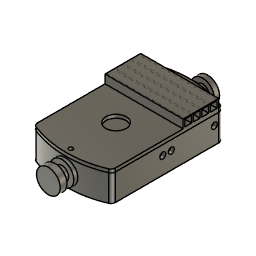
Case (Autodesk Fusion 360 design; units mm, degrees)
Autodesk Fusion 360 part; units mm, degrees
note: some values were not read from the file. Set by a fixed rule: which sketch regions a step uses.
sketch "Boceto1" plane through (0, 0, 0) normal (0, 0, 1) x (1, 0, 0)
  circle A0 centre (-5.9, 16.8256) radius 0.6
  line L0 (10.4, -15.2481) -> (-10.4, -15.2481)
  line L1 (-10.4, 15.5519) -> (-4.2071, 15.5519)
  circle A1 centre (5.9, 16.8256) radius 0.6
  spline S0 degree 3 poles (10.7171, -16.1976) (9.0911, -16.9299) (7.3492, -17.4466) (3.7858, -18.1418) (1.8989, -18.3158) (-4.1389, -18.2732) (-7.7725, -17.3263) (-10.6417, -16.2266) knots -1.732785 -1.732785 -1.732785 -1.732785 -1.337909 -1.337909 -0.921833 -0.921833 0 0 0 0
  line L2 (4.1929, 15.5519) -> (10.4, 15.5519)
  circle A2 centre (0, -16.6178) radius 0.6
  arc A3 (10.7171, -16.1976) -> (11.5, -15.0181) centre (10.22, -15.0181) ccw
  arc A4 (-11.5, -15.0181) -> (-10.6417, -16.2266) centre (-10.22, -15.0181) ccw
  line L3 (10.4, 15.5519) -> (10.4, -15.2481)
  line L4 (11.5, -15.0181) -> (11.4989, 15.4432)
  line L5 (-11.5011, 15.4432) -> (-11.5, -15.0181)
  line L6 (-10.4, -15.2481) -> (-10.4, 15.5519)
  line L7 (4.1929, 15.5519) -> (-4.2071, 15.5519)
  spline S1 degree 3 poles (-10.7181, 16.6227) (-9.0922, 17.355) (-7.3503, 17.8717) (-3.7869, 18.5669) (-1.9, 18.7409) (4.1378, 18.6983) (7.7714, 17.7514) (10.6407, 16.6517) knots -1.732785 -1.732785 -1.732785 -1.732785 -1.337909 -1.337909 -0.921833 -0.921833 0 0 0 0
  arc A5 (11.4989, 15.4432) -> (10.6407, 16.6517) centre (10.2189, 15.4432) ccw
  arc A6 (-10.7181, 16.6227) -> (-11.5011, 15.4432) centre (-10.2211, 15.4432) ccw
  point P0 (10.3989, 15.6732)
  point P1 (-10.4011, 15.6732)
  constraint coincident L5.start A6.end
  constraint coincident L4.end A5.start
extrude "Extruir1" add sketch "Boceto1" along normal blind 5.6 makes body 1
sketch "Boceto3" plane through (0, 0, 0) normal (0, 0, 1) x (1, 0, 0)
  spline S0 degree 3 poles (-10.7181, 16.6227) (-9.0922, 17.355) (-7.3503, 17.8717) (-3.7869, 18.5669) (-1.9, 18.7409) (4.1378, 18.6983) (7.7714, 17.7514) (10.6407, 16.6517) knots -1.732785 -1.732785 -1.732785 -1.732785 -1.337909 -1.337909 -0.921833 -0.921833 0 0 0 0
  line L0 (-11.5011, 15.4432) -> (-11.5, -15.0181)
  line L1 (11.5, -15.0181) -> (11.4989, 15.4432)
  spline S1 degree 3 poles (10.7171, -16.1976) (9.0911, -16.9299) (7.3492, -17.4466) (3.7858, -18.1418) (1.8989, -18.3158) (-4.1389, -18.2732) (-7.7725, -17.3263) (-10.6417, -16.2266) knots -1.732785 -1.732785 -1.732785 -1.732785 -1.337909 -1.337909 -0.921833 -0.921833 0 0 0 0
  arc A0 (-11.5, -15.0181) -> (-10.6417, -16.2266) centre (-10.22, -15.0181) ccw
  arc A1 (10.7171, -16.1976) -> (11.5, -15.0181) centre (10.22, -15.0181) ccw
  arc A2 (11.4989, 15.4432) -> (10.6407, 16.6517) centre (10.2189, 15.4432) ccw
  arc A3 (-10.7181, 16.6227) -> (-11.5011, 15.4432) centre (-10.2211, 15.4432) ccw
  point P0 (10.3989, 15.6732)
  point P1 (-10.4011, 15.6732)
  constraint coincident L0.start A3.end
  constraint coincident L1.end A2.start
extrude "Extruir2" add sketch "Boceto3" against normal blind 2.2 bodies 1
sketch "Boceto4" plane through (0, 0, 5.6) normal (0, 0, 1) x (-1, 0, 0)
  circle A0 centre (0, 16.6178) radius 0.6
  circle A1 centre (-5.9, -16.8256) radius 0.6
  circle A2 centre (5.9, -16.8256) radius 0.6
  line L0 (10.4, -15.5519) -> (-10.4, -15.5519)
  line L1 (-10.4, -15.5519) -> (-10.4, 15.2481)
  line L2 (-10.4, 15.2481) -> (10.4, 15.2481)
  line L3 (10.4, 15.2481) -> (10.4, -15.5519)
  arc A3 (-10.7171, 16.1976) -> (-11.5, 15.0181) centre (-10.22, 15.0181) ccw
  line L4 (-11.5, 15.0181) -> (-11.4989, -15.4432)
  line L5 (11.5011, -15.4432) -> (11.5, 15.0181)
  arc A4 (11.5, 15.0181) -> (10.6417, 16.2266) centre (10.22, 15.0181) ccw
  spline S0 degree 3 poles (10.6417, 16.2266) (7.7725, 17.3263) (4.1389, 18.2732) (-1.8989, 18.3158) (-3.7858, 18.1418) (-7.3492, 17.4466) (-9.0911, 16.9299) (-10.7171, 16.1976) knots 0 0 0 0 0.921833 0.921833 1.337909 1.337909 1.732785 1.732785 1.732785 1.732785
  line L6 (0, 16.6178) -> (0, 18.3024) construction
  line L7 (0, 18.3024) -> (0, 23.3024) construction
  line L8 (0, 23.3024) -> (5.4941, 23.3024) construction
  line L9 (0, -15.5519) -> (0, -18.7081) construction
  line L10 (0, -18.7081) -> (0, -23.7081) construction
  line L11 (0, -23.7081) -> (4.3514, -23.7081) construction
  arc A5 (-11.4989, -15.4432) -> (-10.6407, -16.6517) centre (-10.2189, -15.4432) ccw
  spline S1 degree 3 poles (-10.6407, -16.6517) (-7.7714, -17.7514) (-4.1378, -18.6983) (1.9, -18.7409) (3.7869, -18.5669) (7.3503, -17.8717) (9.0922, -17.355) (10.7181, -16.6227) knots 0 0 0 0 0.921833 0.921833 1.337909 1.337909 1.732785 1.732785 1.732785 1.732785
  arc A6 (10.7181, -16.6227) -> (11.5011, -15.4432) centre (10.2211, -15.4432) ccw
  dimension "d6" = 5
  dimension "d7" = 5
  constraint coincident A0.centre L6.start
  constraint coincident S0 L6.end
  constraint vertical L6
  constraint parallel L6 L7
  constraint perpendicular L7 L8
  constraint midpoint L0 L9.start
  constraint perpendicular L0 L9
  constraint perpendicular L0 L10
  constraint perpendicular L10 L11
  measures "d6" distance of L6.end L7.end
  measures "d7" distance of L9.end L10.end
ref_plane "PlanoDeObra1" through (-2.747, -23.3024, 5.6) normal (0, 1, 0) x (-1, 0, 0)
ref_plane "PlanoDeObra2" through (-2.1757, 23.7081, 5.6) normal (0, 1, 0) x (-1, 0, 0)
sketch "Boceto5" plane through (0, -23.3024, 0) normal (0, 1, 0) x (1, 0, 0)
  line L0 (10.7171, 2.2) -> (10.7171, -5.6)
  line L1 (-10.6417, -5.6) -> (10.7171, -5.6)
  line L2 (-10.6417, -5.6) -> (-10.6417, 2.2)
  line L3 (10.7171, 2.2) -> (-10.6417, 2.2)
  line L4 (-10.6417, -5.6) -> (10.7171, 2.2) construction
  line L5 (-10.6417, 2.2) -> (10.7171, -5.6) construction
  circle A0 centre (0.0377, -1.7) radius 3.5
  dimension "d10" = 7
  constraint coincident L1.start L2.start
  constraint coincident L0.start L3.start
  constraint coincident L2.end L3.end
  constraint coincident L0.end L1.end
  constraint midpoint L4 A0.centre
  measures "d10" diameter of A0
extrude "Extruir3" add sketch "Boceto5" along normal up to surface contours A0 end surface at (-2.3988, -18.1819, 2.4889) on bodies 1 bodies 1
sketch "Boceto6" plane through (0, 23.7081, 0) normal (0, 1, 0) x (1, 0, 0)
  line L0 (4.1929, 0) -> (-4.2071, 2.2) construction
  line L1 (4.1929, 2.2) -> (-4.2071, 0) construction
  line L2 (-10.7181, 2.2) -> (-10.7181, -5.6)
  line L3 (10.6407, -5.6) -> (-10.7181, -5.6)
  line L4 (10.6407, -5.6) -> (10.6407, 2.2)
  line L5 (-10.7181, 2.2) -> (10.6407, 2.2)
  line L6 (10.6407, -5.6) -> (-10.7181, 2.2) construction
  line L7 (10.6407, 2.2) -> (-10.7181, -5.6) construction
  circle A0 centre (-0.0387, -1.7) radius 3.5
  dimension "d42" = 7
  constraint coincident L3.start L4.start
  constraint coincident L2.start L5.start
  constraint coincident L4.end L5.end
  constraint coincident L2.end L3.end
  constraint midpoint L6 A0.centre
  measures "d42" diameter of A0
extrude "Extruir4" add sketch "Boceto6" against normal up to surface (8.1561 mm away) contours A0 bodies 1
sketch "Boceto7" plane through (0, 0, -2.2) normal (0, 0, -1) x (1, 0, 0)
  line L0 (11.4989, -15.4432) -> (11.5, 15.0181)
  arc A0 (11.5, 15.0181) -> (10.7171, 16.1976) centre (10.22, 15.0181) ccw
  spline S0 degree 3 poles (10.7171, 16.1976) (9.0911, 16.9299) (7.3492, 17.4466) (3.7858, 18.1418) (1.8989, 18.3158) (-4.1389, 18.2732) (-7.7725, 17.3263) (-10.6417, 16.2266) knots -1.732785 -1.732785 -1.732785 -1.732785 -1.337909 -1.337909 -0.921833 -0.921833 0 0 0 0
  arc A1 (-10.6417, 16.2266) -> (-11.5, 15.0181) centre (-10.22, 15.0181) ccw
  line L1 (-11.5, 15.0181) -> (-11.5011, -15.4432)
  arc A2 (-5.775, -6.6) -> (-5.775, -15) centre (-5.775, -10.8) ccw
  line L2 (5.775, 4.2) -> (-5.775, 4.2)
  arc A3 (5.775, -4.2) -> (5.775, 4.2) centre (5.775, 0) ccw
  arc A4 (5.775, -15) -> (5.775, -6.6) centre (5.775, -10.8) ccw
  line L3 (5.775, 15) -> (-5.775, 15)
  arc A5 (5.775, 6.6) -> (5.775, 15) centre (5.775, 10.8) ccw
  line L4 (-5.775, -15) -> (5.775, -15)
  arc A6 (-5.775, 4.2) -> (-5.775, -4.2) centre (-5.775, 0) ccw
  line L5 (-5.775, 6.6) -> (5.775, 6.6)
  arc A7 (-5.775, 15) -> (-5.775, 6.6) centre (-5.775, 10.8) ccw
  line L6 (-5.775, -4.2) -> (5.775, -4.2)
  line L7 (5.775, -6.6) -> (-5.775, -6.6)
  arc A8 (-11.5011, -15.4432) -> (-10.7181, -16.6227) centre (-10.2211, -15.4432) ccw
  spline S1 degree 3 poles (-10.7181, -16.6227) (-9.0922, -17.355) (-7.3503, -17.8717) (-3.7869, -18.5669) (-1.9, -18.7409) (4.1378, -18.6983) (7.7714, -17.7514) (10.6407, -16.6517) knots -1.732785 -1.732785 -1.732785 -1.732785 -1.337909 -1.337909 -0.921833 -0.921833 0 0 0 0
  arc A9 (10.6407, -16.6517) -> (11.4989, -15.4432) centre (10.2189, -15.4432) ccw
sketch "Boceto8" plane through (0, 0, 0) normal (0, 0, 1) x (-1, 0, 0)
  line L0 (10.4, -15.5519) -> (10.4, 15.2481)
  line L1 (10.4, 15.2481) -> (-10.4, 15.2481)
  line L2 (-10.4, 15.2481) -> (-10.4, -15.5519)
  line L3 (-10.4, -15.5519) -> (10.4, -15.5519)
  arc A0 (-1, 1.0002) -> (-1, -0.9998) centre (-1, 0.0002) ccw
  line L4 (3, 1.0002) -> (3, 1.0002)
  arc A1 (-1, 1.0002) -> (-1, -0.9998) centre (-1, 0.0002) ccw
  line L5 (-1, 11.7998) -> (3, 11.7998)
  line L6 (3, -11.7997) -> (-1, -11.7997)
  arc A2 (-1, -9.7997) -> (-1, -11.7997) centre (-1, -10.7997) ccw
  arc A3 (3, 9.7998) -> (3, 11.7998) centre (3, 10.7998) ccw
  arc A4 (3, -0.9998) -> (3, 1.0002) centre (3, 0.0002) ccw
  line L7 (-1, -11.7997) -> (3, -11.7997)
  line L8 (3, 9.7998) -> (-1, 9.7998)
  line L9 (-1, -0.9998) -> (3, -0.9998)
  arc A5 (3, -11.7997) -> (3, -9.7997) centre (3, -10.7997) ccw
  line L10 (3, -0.9998) -> (-1, -0.9998)
  line L11 (3, -9.7997) -> (-1, -9.7997)
  arc A6 (-1, 11.7998) -> (-1, 9.7998) centre (-1, 10.7998) ccw
  arc A7 (3, -0.9998) -> (3, 1.0002) centre (3, 0.0002) ccw
  arc A8 (3, -11.7997) -> (3, -9.7997) centre (3, -10.7997) ccw
  line L12 (-1, 1.0002) -> (3, 1.0002)
  arc A9 (-1, -9.7997) -> (-1, -11.7997) centre (-1, -10.7997) ccw
  line L13 (-1, 0.8945) -> (-1, 0.8945)
  line L14 (-1, 1.8945) -> (-1, 1.8945)
  line L15 (3, 1.8945) -> (3, 1.8945)
  line L16 (-1, -9.7997) -> (3, -9.7997)
  line L17 (3, 0.8945) -> (3, 0.8945)
extrude "Extruir5" cut sketch "Boceto8" against normal blind 1 contours A0 A1 A4 L9 L10 A7 L12 | L5 A3 L8 A6 | L6 A2 L7 A5 L11 A8 A9 L16 bodies 1
extrude "Extruir6" cut sketch "Boceto7" against normal blind 1.2 contours A2 A4 L4 L7 | L2 A3 A6 L6 | L3 A5 L5 A7 bodies 1
ref_plane "PlanoDeObra3" through (-0.0005, 0.2126, 5.6) normal (0, 0, 1) x (1, 0, 0)
sketch "Boceto9" plane through (0, 0, 5.6) normal (0, 0, 1) x (1, 0, 0)
  arc A0 (-10.7181, 16.6227) -> (-11.5011, 15.4432) centre (-10.2211, 15.4432) ccw
  arc A1 (11.4989, 15.4432) -> (10.6407, 16.6517) centre (10.2189, 15.4432) ccw
  line L0 (-10.4, 15.5519) -> (-4.2071, 15.5519)
  line L1 (-11.5011, 15.4432) -> (-11.5, -15.0181)
  circle A2 centre (-5.9, 16.8256) radius 0.6
  arc A3 (10.7171, -16.1976) -> (11.5, -15.0181) centre (10.22, -15.0181) ccw
  line L2 (11.5, -15.0181) -> (11.4989, 15.4432)
  spline S0 degree 3 poles (-10.7181, 16.6227) (-9.0922, 17.355) (-7.3503, 17.8717) (-3.7869, 18.5669) (-1.9, 18.7409) (4.1378, 18.6983) (7.7714, 17.7514) (10.6407, 16.6517) knots -1.732785 -1.732785 -1.732785 -1.732785 -1.337909 -1.337909 -0.921833 -0.921833 0 0 0 0
  line L3 (10.4, 15.5519) -> (10.4, -15.2481)
  circle A4 centre (0, -16.6178) radius 0.6
  line L4 (4.1929, 15.5519) -> (10.4, 15.5519)
  line L5 (-10.4, -15.2481) -> (-10.4, 15.5519)
  line L6 (4.1929, 15.5519) -> (-4.2071, 15.5519)
  spline S1 degree 3 poles (10.7171, -16.1976) (9.0911, -16.9299) (7.3492, -17.4466) (3.7858, -18.1418) (1.8989, -18.3158) (-4.1389, -18.2732) (-7.7725, -17.3263) (-10.6417, -16.2266) knots -1.732785 -1.732785 -1.732785 -1.732785 -1.337909 -1.337909 -0.921833 -0.921833 0 0 0 0
  arc A5 (-11.5, -15.0181) -> (-10.6417, -16.2266) centre (-10.22, -15.0181) ccw
  line L7 (10.4, -15.2481) -> (-10.4, -15.2481)
  circle A6 centre (5.9, 16.8256) radius 0.6
  point P0 (10.3989, 15.6732)
  point P1 (-10.4011, 15.6732)
  constraint coincident A0.end L1.start
  constraint coincident A1.start L2.end
extrude "Extruir7" add sketch "Boceto9" along normal blind 1 separate body contours A0 A1 L1 A3 L2 S0 S1 A5 | L0 L3 L4 L5 L6 L7 makes body 2
sketch "Boceto10" plane through (0, 0, 6.6) normal (0, 0, 1) x (-1, 0, 0)
  circle A0 centre (-5.9, -16.8256) radius 0.6
  circle A1 centre (0, 16.6178) radius 0.6
  circle A2 centre (5.9, -16.8256) radius 0.6
  arc A3 (10.7181, -16.6227) -> (11.5011, -15.4432) centre (10.2211, -15.4432) ccw
  line L0 (11.5011, -15.4432) -> (11.5, 15.0181)
  arc A4 (11.5, 15.0181) -> (10.6417, 16.2266) centre (10.22, 15.0181) ccw
  spline S0 degree 3 poles (10.6417, 16.2266) (7.7725, 17.3263) (4.1389, 18.2732) (-1.8989, 18.3158) (-3.7858, 18.1418) (-7.3492, 17.4466) (-9.0911, 16.9299) (-10.7171, 16.1976) knots 0 0 0 0 0.921833 0.921833 1.337909 1.337909 1.732785 1.732785 1.732785 1.732785
  arc A5 (-10.7171, 16.1976) -> (-11.5, 15.0181) centre (-10.22, 15.0181) ccw
  line L1 (-11.5, 15.0181) -> (-11.4989, -15.4432)
  arc A6 (-11.4989, -15.4432) -> (-10.6407, -16.6517) centre (-10.2189, -15.4432) ccw
  spline S1 degree 3 poles (-10.6407, -16.6517) (-7.7714, -17.7514) (-4.1378, -18.6983) (1.9, -18.7409) (3.7869, -18.5669) (7.3503, -17.8717) (9.0922, -17.355) (10.7181, -16.6227) knots 0 0 0 0 0.921833 0.921833 1.337909 1.337909 1.732785 1.732785 1.732785 1.732785
  line L2 (0, 16.6178) -> (0, 3.3178) construction
  circle A7 centre (0, 3.3178) radius 3
  dimension "d43" = 13.3
  dimension "d44" = 6
  constraint coincident A1.centre L2.start
  constraint vertical L2
  constraint coincident L2.end A7.centre
  measures "d43" distance of A1.centre L2.end
  measures "d44" diameter of A7
extrude "Extruir8" cut sketch "Boceto10" against normal through all contours A7 bodies 2
sketch "Boceto11" plane through (11.4995, 0.0004, 0) normal (1, 0.000035, 0) x (-0.000035, 1, 0)
  line L0 (-15.0185, 5.6) -> (-15.0185, -2.2)
  line L1 (-15.0185, -2.2) -> (15.4428, -2.2)
  line L2 (15.4428, -2.2) -> (15.4428, 0) construction
  line L3 (15.4428, 0) -> (-15.0185, 0) construction
  line L4 (-15.0185, 5.6) -> (15.4428, 0) construction
  line L5 (-15.0185, 0) -> (15.4219, 5.6) construction
  line L6 (0.2122, 2.8) -> (0.2122, 0) construction
  line L7 (0.2122, 2.8) -> (1.4622, 2.8) construction
  line L8 (0.2122, 2.8) -> (-1.0378, 2.8) construction
  circle A0 centre (1.4622, 2.8) radius 0.9
  circle A1 centre (-1.0378, 2.8) radius 0.9
  line L9 (15.4428, -2.2) -> (15.4428, 5.6)
  line L10 (15.4428, 5.6) -> (-15.0185, 5.6)
  dimension "d26" = 2.2
  dimension "d27" = 1.25
  dimension "d28" = 1.25
  dimension "d29" = 1.8
  dimension "d30" = 1.8
  constraint coincident L1.end L2.start
  constraint perpendicular L1 L2
  constraint coincident L0 L3.end
  constraint perpendicular L0 L3
  constraint coincident L0.start L4.start
  constraint midpoint L4 L6.start
  constraint midpoint L3 L6.end
  constraint perpendicular L6 L7
  constraint perpendicular L6 L8
  constraint coincident L7.end A0.centre
  constraint coincident L8.end A1.centre
  measures "d26" distance of L1.end L2.end
  measures "d27" distance of L6.start L7.end
  measures "d28" distance of L6.start L8.end
  measures "d29" diameter of A0
  measures "d30" diameter of A1
extrude "Extruir9" cut sketch "Boceto11" against normal blind 23 contours A0 | A1 bodies 1
sketch "Boceto12" plane through (11.4995, 0.0004, 0) normal (1, 0.000035, 0) x (-0.000035, 1, 0)
  circle A0 centre (-1.0378, 2.8) radius 0.9
  circle A1 centre (1.4622, 2.8) radius 0.9
  line L0 (15.4428, 5.6) -> (-15.0185, 5.6)
  line L1 (-15.0185, 5.6) -> (-15.0185, -2.2)
  line L2 (-15.0181, 5.6) -> (-15.0181, -2.2)
  line L3 (15.4219, 5.6) -> (-15.0181, 5.6)
  line L4 (15.4219, -2.2) -> (15.4219, 0) construction
  line L5 (15.4219, 0) -> (-15.0181, 0) construction
  line L6 (15.4219, -2.2) -> (15.4219, 5.6)
  line L7 (-15.0181, -2.2) -> (15.4219, -2.2)
  line L8 (1.4622, 2.8) -> (15.4219, 2.8) construction
  line L9 (15.4219, 2.8) -> (14.1719, 2.8) construction
  circle A2 centre (14.1719, 2.8) radius 0.9
  line L10 (15.4428, -2.2) -> (15.4428, 5.6)
  line L11 (-15.0185, -2.2) -> (15.4428, -2.2)
  dimension "d33" = 2.2
  dimension "d38" = 1.25
  dimension "d39" = 1.8
  constraint coincident L4.start L6.start
  constraint perpendicular L4 L7
  constraint coincident L5.end L2
  constraint perpendicular L2 L5
  constraint coincident A1.centre L8.start
  constraint coincident L6 L8.end
  constraint perpendicular L6 L8
  constraint perpendicular L6 L9
  constraint coincident L9.end A2.centre
  measures "d33" distance of L4.start L4.end
  measures "d38" distance of L8.end L9.end
  measures "d39" diameter of A2
extrude "Extruir10" cut sketch "Boceto12" against normal blind 3 contours A2 bodies 1
ref_plane "PlanoDeObra4" through (0.0377, -20.3024, 1.7) normal (0, -1, 0) x (-1, 0, 0)
sketch "Boceto13" plane through (0, -20.3024, 0) normal (0, -1, 0) x (-1, 0, 0)
  circle A0 centre (-0.0377, -1.7) radius 3.5
  circle A1 centre (-0.0377, -1.7) radius 3.5
  circle A2 centre (-0.0377, -1.7) radius 2
  dimension "d46" = 4
  constraint concentric A0 A1
  constraint concentric A0 A2
  measures "d46" diameter of A2
extrude "Extruir11" cut sketch "Boceto13" along normal mid plane 2 bodies 1
ref_plane "PlanoDeObra5" through (-0.0387, 21.2081, 1.7) normal (0, 1, 0) x (1, 0, 0)
sketch "Boceto16" plane through (0, 21.2081, 0) normal (0, 1, 0) x (1, 0, 0)
  circle A0 centre (-0.0387, -1.7) radius 3.5
  circle A1 centre (-0.0387, -1.7) radius 3.5
  circle A2 centre (-0.0387, -1.7) radius 2
  dimension "d50" = 4
  constraint concentric A0 A1
  constraint concentric A1 A2
  measures "d50" diameter of A2
extrude "Extruir12" cut sketch "Boceto16" along normal mid plane 2 bodies 1
sketch "Boceto18" plane through (0, 0, 6.6) normal (0, 0, 1) x (-1, 0, 0)
  circle A0 centre (0, 3.3178) radius 3
  circle A1 centre (-5.9, -16.8256) radius 0.6
  circle A2 centre (0, 16.6178) radius 0.6
  circle A3 centre (5.9, -16.8256) radius 0.6
  arc A4 (10.7181, -16.6227) -> (11.5011, -15.4432) centre (10.2211, -15.4432) ccw
  line L0 (11.5011, -15.4432) -> (11.5, 15.0181)
  arc A5 (11.5, 15.0181) -> (10.6417, 16.2266) centre (10.22, 15.0181) ccw
  spline S0 degree 3 poles (10.6417, 16.2266) (7.7725, 17.3263) (4.1389, 18.2732) (-1.8989, 18.3158) (-3.7858, 18.1418) (-7.3492, 17.4466) (-9.0911, 16.9299) (-10.7171, 16.1976) knots 0 0 0 0 0.921833 0.921833 1.337909 1.337909 1.732785 1.732785 1.732785 1.732785
  arc A6 (-10.7171, 16.1976) -> (-11.5, 15.0181) centre (-10.22, 15.0181) ccw
  line L1 (-11.5, 15.0181) -> (-11.4989, -15.4432)
  arc A7 (-11.4989, -15.4432) -> (-10.6407, -16.6517) centre (-10.2189, -15.4432) ccw
  spline S1 degree 3 poles (-10.6407, -16.6517) (-7.7714, -17.7514) (-4.1378, -18.6983) (1.9, -18.7409) (3.7869, -18.5669) (7.3503, -17.8717) (9.0922, -17.355) (10.7181, -16.6227) knots 0 0 0 0 0.921833 0.921833 1.337909 1.337909 1.732785 1.732785 1.732785 1.732785
  line L2 (-11.4989, -15.4432) -> (11.5011, -15.4432)
  line L3 (0.0011, -15.4432) -> (0.0011, -13.9432)
  line L4 (0.0011, -13.9432) -> (0.0011, -11.4432)
  line L5 (0.0011, -11.4432) -> (0.0011, -8.9432)
  line L6 (0.0011, -8.9432) -> (0.0011, -6.4432)
  line L7 (0.0011, -6.4432) -> (0.0011, -4.9432)
  line L8 (0.0011, -4.9432) -> (11.5007, -4.9428)
  line L9 (11.5007, -4.9428) -> (11.5011, -15.4432)
  line L10 (0.0011, -4.9432) -> (-11.4993, -4.9436)
  line L11 (-11.4993, -4.9436) -> (-11.4989, -15.4432)
  dimension "d53" = 1.5
  dimension "d54" = 2.5
  dimension "d55" = 2.5
  dimension "d56" = 2.5
  dimension "d57" = 1.5
  constraint coincident L1.end A7.start
  constraint coincident A4.end L0.start
  constraint midpoint L2 L3.start
  constraint perpendicular L2 L3
  constraint parallel L3 L4
  constraint parallel L4 L5
  constraint parallel L5 L6
  constraint parallel L6 L7
  constraint coincident L0 L8.end
  constraint perpendicular L0 L8
  constraint coincident L1 L10.end
  constraint perpendicular L1 L10
  constraint perpendicular L10 L11
  measures "d53" distance of L3.start L3.end
  measures "d54" distance of L3.end L4.end
  measures "d55" distance of L4.end L5.end
  measures "d56" distance of L5.end L6.end
  measures "d57" distance of L6.end L7.end
extrude "Extruir13" add sketch "Boceto18" along normal blind 2.5 contours L0 L2 L3 L4 L5 L6 L7 L8 L9 | L1 L2 L3 L4 L5 L6 L7 L10 L11 bodies 2
sketch "Boceto19" plane through (11.4995, 0.0004, 0) normal (1, 0.000035, 0) x (-0.000035, 1, 0)
  line L0 (-15.0185, 5.6) -> (15.4428, 5.6)
  line L1 (15.4428, 5.6) -> (15.4428, 6.6)
  line L2 (15.4428, 6.6) -> (15.4428, 9.1)
  line L3 (15.4428, 9.1) -> (4.9432, 9.1)
  line L4 (4.9432, 9.1) -> (4.9432, 6.6)
  line L5 (4.9432, 6.6) -> (-15.0185, 6.6)
  line L6 (-15.0185, 6.6) -> (-15.0185, 5.6)
  line L7 (15.4428, 6.6) -> (4.9432, 6.6) construction
  line L8 (15.4428, 6.6) -> (15.4428, 9.1) construction
  line L9 (4.9432, 9.1) -> (4.9432, 6.6) construction
  line L10 (15.4428, 9.1) -> (4.9432, 9.1) construction
  line L11 (15.4428, 7.85) -> (13.9428, 7.85) construction
  line L12 (13.9428, 7.85) -> (11.4428, 7.85) construction
  line L13 (11.4428, 7.85) -> (8.9428, 7.85) construction
  line L14 (8.9428, 7.85) -> (6.4428, 7.85) construction
  line L15 (6.4428, 7.85) -> (5.1928, 7.85) construction
  circle A0 centre (6.4428, 7.85) radius 0.9 construction
  circle A1 centre (8.9428, 7.85) radius 0.9 construction
  circle A2 centre (11.4428, 7.85) radius 0.9 construction
  circle A3 centre (13.9428, 7.85) radius 0.9 construction
  line L16 (7.4428, 6.85) -> (5.4428, 6.85)
  line L17 (5.4428, 6.85) -> (5.4428, 8.85)
  line L18 (5.4428, 8.85) -> (7.4428, 8.85)
  line L19 (7.4428, 8.85) -> (7.4428, 6.85)
  line L20 (7.4428, 6.85) -> (5.4428, 8.85) construction
  line L21 (5.4428, 6.85) -> (7.4428, 8.85) construction
  line L22 (9.9428, 6.85) -> (7.9428, 6.85)
  line L23 (7.9428, 6.85) -> (7.9428, 8.85)
  line L24 (7.9428, 8.85) -> (9.9428, 8.85)
  line L25 (9.9428, 8.85) -> (9.9428, 6.85)
  line L26 (9.9428, 6.85) -> (7.9428, 8.85) construction
  line L27 (7.9428, 6.85) -> (9.9428, 8.85) construction
  line L28 (12.4428, 6.85) -> (10.4428, 6.85)
  line L29 (10.4428, 6.85) -> (10.4428, 8.85)
  line L30 (10.4428, 8.85) -> (12.4428, 8.85)
  line L31 (12.4428, 8.85) -> (12.4428, 6.85)
  line L32 (12.4428, 6.85) -> (10.4428, 8.85) construction
  line L33 (10.4428, 6.85) -> (12.4428, 8.85) construction
  line L34 (14.9428, 6.85) -> (12.9428, 6.85)
  line L35 (12.9428, 6.85) -> (12.9428, 8.85)
  line L36 (12.9428, 8.85) -> (14.9428, 8.85)
  line L37 (14.9428, 8.85) -> (14.9428, 6.85)
  line L38 (14.9428, 6.85) -> (12.9428, 8.85) construction
  line L39 (12.9428, 6.85) -> (14.9428, 8.85) construction
  point P0 (6.4428, 7.85)
  point P1 (8.9428, 7.85)
  point P2 (11.4428, 7.85)
  point P3 (13.9428, 7.85)
  dimension "d60" = 1.5
  dimension "d61" = 2.5
  dimension "d62" = 2.5
  dimension "d63" = 2.5
  dimension "d64" = 1.25
  dimension "d65" = 1.8
  dimension "d66" = 1.8
  dimension "d67" = 1.8
  dimension "d68" = 1.8
  dimension "d69" = 2
  dimension "d70" = 2
  dimension "d71" = 2
  dimension "d72" = 2
  dimension "d73" = 2
  dimension "d74" = 2
  dimension "d75" = 2
  dimension "d76" = 2
  constraint coincident L1.end L2.start
  constraint coincident L4.end L5.start
  constraint coincident L2.end L3.start
  constraint coincident L3.end L4.start
  constraint midpoint L2 L11.start
  constraint perpendicular L9 L11
  constraint parallel L11 L12
  constraint parallel L12 L13
  constraint parallel L13 L14
  constraint perpendicular L9 L15
  constraint coincident P0 L14.end
  constraint coincident P1 L13.end
  constraint coincident P2 L12.end
  constraint coincident P3 L11.end
  constraint horizontal L16
  constraint perpendicular L16 L17
  constraint parallel L16 L18
  constraint parallel L17 L19
  constraint coincident L20 P0
  constraint coincident L21 P0
  constraint horizontal L22
  constraint perpendicular L22 L23
  constraint parallel L22 L24
  constraint parallel L23 L25
  constraint coincident L26 P1
  constraint coincident L27 P1
  constraint horizontal L28
  constraint perpendicular L28 L29
  constraint parallel L28 L30
  constraint parallel L29 L31
  constraint coincident L32 P2
  constraint coincident L33 P2
  constraint horizontal L34
  constraint perpendicular L34 L35
  constraint parallel L34 L36
  constraint parallel L35 L37
  constraint coincident L38 P3
  constraint coincident L39 P3
  measures "d60" distance of L11.start P3
  measures "d61" distance of P3 P2
  measures "d62" distance of P2 P1
  measures "d63" distance of P1 P0
  measures "d64" distance of P0 L15.end
  measures "d65" diameter of A0
  measures "d66" diameter of A1
  measures "d67" diameter of A2
  measures "d68" diameter of A3
  measures "d69" distance of L17.end L18.end
  measures "d70" distance of L16.end L17.end
  measures "d71" distance of L23.end L24.end
  measures "d72" distance of L22.end L23.end
  measures "d73" distance of L29.end L30.end
  measures "d74" distance of L28.end L29.end
  measures "d75" distance of L35.end L36.end
  measures "d76" distance of L34.end L35.end
extrude "Extruir14" cut sketch "Boceto19" against normal through all contours L16 L17 L18 L19 | L22 L23 L24 L25 | L28 L29 L30 L31 | L34 L35 L36 L37 bodies 2
equation "d27 = ( 2.5 / 2 ) * 1 mm"
equation "d28 = ( 2.5 / 2 ) * 1 mm"
equation "d38 = ( 2.5 / 2 ) * 1 mm"
named bodies: "Case", "Tapa"
